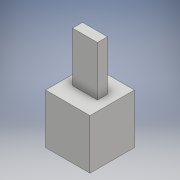
# Autodesk Inventor part: PulleySocket
Saved by Autodesk Inventor 2017 (Build 210142000, 142)
## iProperties
Created: 2017-02-11
Part Number: PulleySocket
Material: Generic
Document SubType Name: Modeling
Designer: aribu
Density: 1 g/cm^3
Appearance: Default
Author: aribu
Autodesk Inventor part; units mm, degrees
ref_plane "YZ Plane" through (0, 0, 0) normal (1, 0, 0) x (0, 1, 0)
ref_plane "XZ Plane" through (0, 0, 0) normal (0, 1, 0) x (-1, 0, 0)
ref_plane "XY Plane" through (0, 0, 0) normal (0, 0, 1) x (1, 0, 0)
sketch "Sketch1" plane through (0, 0, 0) normal (0, 0, 1) x (1, 0, 0)
  line L0 (-4.45, 4.45) -> (4.45, 4.45)
  line L1 (4.45, 4.45) -> (4.45, -4.45)
  line L2 (4.45, -4.45) -> (-4.45, -4.45)
  line L3 (-4.45, -4.45) -> (-4.45, 4.45)
  point P0 (0, 0)
  dimension "d0" = 8.9
  dimension "d1" = 8.9
  dimension "d2" = 4.45
  dimension "d3" = 4.45
  constraints: 8 end point, 2 parallel, 1 horizontal, 1 perpendicular
  measures "d0" distance of L0.start L0.end
  measures "d1" distance of L0.end L1.end
  measures "d2" distance from line of L0 point (0, 0)
  measures "d3" distance from line of point (0, 0) L1
extrude "Extrusion1" add sketch "Sketch1" along normal blind 10
sketch "Sketch2" plane through (0, 0, 10) normal (0, 0, 1) x (1, 0, 0)
  line L0 (-2.5, 1) -> (2.5, 1)
  line L1 (2.5, 1) -> (2.5, -1)
  line L2 (2.5, -1) -> (-2.5, -1)
  line L3 (-2.5, -1) -> (-2.5, 1)
  point P0 (0, 0)
  dimension "d6" = 2
  dimension "d7" = 5
  dimension "d8" = 1
  dimension "d9" = 2.5
  constraints: 8 end point, 2 parallel, 1 horizontal, 1 perpendicular
  measures "d6" distance of L0.end L1.end
  measures "d7" distance of L0.start L0.end
  measures "d8" distance from line of L0 point (0, 0)
  measures "d9" distance from line of L1 point (0, 0)
extrude "Extrusion2" add sketch "Sketch2" along normal blind 10
equation "\"d1\" = d0"
equation "\"d2\" = 0.5 * d0"
equation "\"d3\" = 0.5 * d0"
equation "\"d8\" = 0.5 * d6"
equation "\"d9\" = 0.5 * d7"
body "Solid1"
